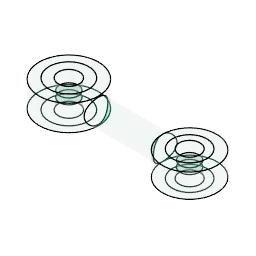
ConnectingBracketV3_v2 (Autodesk Fusion 360 design; units mm, degrees)
Autodesk Fusion 360 part; units mm, degrees
note: some values were not read from the file. Chosen so that the rebuilt part matches the saved one: which bodies a step acts on.
sketch "Sketch1" plane through (0, 0, 0) normal (0, 0, 1) x (1, 0, 0)
  line L0 (0, 0) -> (-12.25, 0) construction
  circle A0 centre (-12.25, 0) radius 0.95
  circle A1 centre (0, 0) radius 0.95
  line L1 (-12.25, 0) -> (-12.25, 0.95) construction
  line L2 (-12.25, 0.95) -> (-12.25, 3) construction
  circle A2 centre (-12.25, 0) radius 3
  line L3 (0, 0) -> (0, 0.95) construction
  line L4 (0, 0.95) -> (0, 2.75) construction
  circle A3 centre (0, 0) radius 2.75
  line L5 (-12.65, 0) -> (-0.95, 0)
  point P0 (-8.279, 0)
  dimension "d9" = 12.25
  dimension "d10" = 1.9
  dimension "d11" = 1.9
  dimension "d30" = 5.5
  dimension "d31" = 6
  constraint coincident L0.start A1.centre
  constraint horizontal L0
  constraint coincident L0.end A0.centre
  constraint coincident A0 L1.end
  constraint perpendicular L0 L1
  constraint perpendicular L0 L2
  constraint concentric A0 A2
  constraint coincident L2.end A2
  constraint coincident A1 L3.end
  constraint perpendicular L0 L3
  constraint vertical L4
  constraint coincident L4.end A3
  constraint coincident L0 L5.start
  constraint coincident L0 L5.end
  constraint coincident A1 L5.end
  measures "d9" distance of L0.start L0.end
  measures "d10" diameter of A0
  measures "d11" diameter of A1
  measures "d30" diameter of A3
  measures "d31" diameter of A2
extrude "Extrude2" add sketch "Sketch1" along normal blind 2.6 makes body 1 at (2.7363, -0.2738, 0.8667) makes body 2 at (-9.2537, -0.1495, 1.7333)
pipe "Pipe1" add diameter 2.4 path "Sketch1" along L5 separate body makes body 3
move_body "Move1" bodies 3 to x (1, 0, 0) y (0, 1, 0) z (0, 0, 1) at (0, 0, 1.3)
combine "Combine1" operation add target body 1 tool bodies 3 2
extrude "Extrude3" cut sketch "Sketch1" along normal blind 4 contours A0 | A1 bodies 1
chamfer "Chamfer1" distance 0.1 distance2 1 2 edges at (-13.1357, 0.3435, 2.6) (-0.8857, 0.3435, 2.6) measured on face at (-9.9445, -0.149, 2.6) measured on face at (2.1362, 0.1838, 2.6) on bodies 1
chamfer "Chamfer2" distance 1 distance2 0.1 2 edges at (-13.1357, 0.3435, 0) (-0.8857, 0.3435, 0) measured on face at (-11.3047, -0.0946, 1.0667) measured on face at (-0.9453, 0.0946, 0.5667) on bodies 1
chamfer "Chamfer3" distance 1 distance2 0.1 2 edges at (-15.047, -1.0848, 2.6) (-2.5639, -0.9944, 2.6) measured on face at (-9.9112, -0.149, 2.6) measured on face at (2.1731, 0.1366, 2.6) on bodies 1
chamfer "Chamfer4" distance 0.1 distance2 1 2 edges at (-2.5639, -0.9944, 0) (-15.047, -1.0848, 0) measured on face at (-2.3453, -1.436, 1.2754) measured on face at (-9.6708, -1.5323, 1.2738) on bodies 1
delete_face "DeleteFace2" 1 faces at (-10.2951, -1.8138, 2.5333) on bodies 1
delete_face "DeleteFace3" 1 faces at (-10.2951, -1.8138, 0.0667) on bodies 1
move_face "OffsetFaces1" offset 0.1 1 faces at (-9.9151, 0.2012, 0) on bodies 1
move_face "OffsetFaces2" offset 0.1 1 faces at (-9.9151, 0.2012, 2.6) on bodies 1
chamfer "Chamfer5" distance 0.1 distance2 1 1 edges at (-15.047, 1.0848, 2.7) measured on face at (-9.2649, 0.2987, 2.6667) on bodies 1
chamfer "Chamfer6" distance 1 distance2 0.1 1 edges at (-15.047, 1.0848, -0.1) measured on face at (-9.9151, 0.2012, -0.1) on bodies 1
